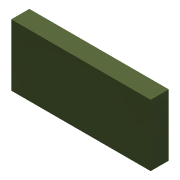
# Autodesk Inventor part: DIGITAL
Saved by Autodesk Inventor 2017 (Build 210142000, 142)
## iProperties
Part Number: DIGITAL
Material: Generisch
Document SubType Name: Modeling
Designer: Werkstatt
Density: 1 g/cm^3
Appearance: 1X08, DIGITAL
Author: Werkstatt
Autodesk Inventor part; units mm, degrees
ref_plane "YZ Plane" through (0, 0, 0) normal (1, 0, 0) x (0, 1, 0)
ref_plane "XZ Plane" through (0, 0, 0) normal (0, 1, 0) x (-1, 0, 0)
ref_plane "XY Plane" through (0, 0, 0) normal (0, 0, 1) x (1, 0, 0)
sketch "1X08, DIGITAL_15" plane through (0, 0, 0) normal (0, 0, 1) x (1, 0, 0)
  line L0 (-1.27, 1.3716) -> (19.05, 1.3716)
  line L1 (19.05, 1.3716) -> (19.05, -1.27)
  line L2 (19.05, -1.27) -> (-1.27, -1.27)
  line L3 (-1.27, -1.27) -> (-1.27, 1.3716)
  constraints: 8 end point
extrude "Extrusion1" add sketch "1X08, DIGITAL_15" along normal blind 9
